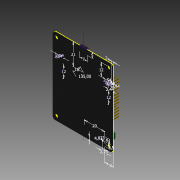
# Autodesk Inventor part: VeyronServoDriver
Saved by Autodesk Inventor 2015 (Build 190159000, 159)
## iProperties
Created: 2015-10-10
Part Number: VeyronServoDriver
Material: Generic
Document SubType Name: Modeling
Designer: styku
Density: 1 g/cm^3
Appearance: Default
Mass: 6.61804 g
Surface Area: 124.511 cm^2
Volume: 6.61804 cm^3
Author: styku
Autodesk Inventor part; units mm, degrees
ref_plane "YZ Plane" through (0, 0, 0) normal (1, 0, 0) x (0, 1, 0)
ref_plane "XZ Plane" through (0, 0, 0) normal (0, 1, 0) x (-1, 0, 0)
ref_plane "XY Plane" through (0, 0, 0) normal (0, 0, 1) x (1, 0, 0)
sketch "Sketch1" plane through (0, 0, 0) normal (0, 1, 0) x (-1, 0, 0)
  line L0 (22, 0) -> (-23, 0) construction
  line L1 (26.5, -36.5) -> (-26.5, -36.5)
  line L2 (-26.5, 36.5) -> (26.5, 36.5)
  line L3 (28.5, 34.5) -> (28.5, -34.5)
  line L4 (-28.5, -34.5) -> (-28.5, 34.5)
  line L5 (0, 32.6896) -> (0, -29) construction
  circle A0 centre (25, 32.5) radius 1.5
  circle A1 centre (-25, 32.5) radius 1.5
  circle A2 centre (25, -32.5) radius 1.5
  circle A3 centre (-25, -32.5) radius 1.5
  arc A4 (28.5, 34.5) -> (26.5, 36.5) centre (26.5, 34.5) ccw
  arc A5 (-26.5, 36.5) -> (-28.5, 34.5) centre (-26.5, 34.5) ccw
  arc A6 (-28.5, -34.5) -> (-26.5, -36.5) centre (-26.5, -34.5) ccw
  arc A7 (26.5, -36.5) -> (28.5, -34.5) centre (26.5, -34.5) ccw
  point P0 (0, 0)
  dimension "d1" = 73
  dimension "d2" = 57
  dimension "d3" = 3
  dimension "d4" = 32.5
  dimension "d5" = 25
  dimension "d6" = 2
  dimension "d7" = 2
  constraints: 12 end point, 8 centre point, 8 point on circle, 8 tangent, 3 symmetric about line, 2 equal radius, 2 horizontal, 2 vertical, 1 parallel, 5 other
  measures "d1" distance between parallel lines of L2 L1
  measures "d2" distance between parallel lines of L4 L3
  measures "d3" diameter of A0
  measures "d4" distance from line of L0 A0.centre
  measures "d5" distance from line of L5 A0.centre
  measures "d6" radius of A4
  measures "d7" radius of A5
extrude "Extrusion1" add sketch "Sketch1" along normal blind 1
sketch "Sketch2" plane through (0, 1, 0) normal (0, 1, 0) x (1, 0, 0)
  circle A0 centre (25, 32.5) radius 1.5 projected
  circle A1 centre (-25, 32.5) radius 1.5 projected
  circle A2 centre (25, -32.5) radius 1.5 projected
  circle A3 centre (-25, -32.5) radius 1.5 projected
  line L0 (-28.5, 34.5) -> (-28.5, -34.5) projected
  arc A4 (-28.5, -34.5) -> (-26.5, -36.5) centre (-26.5, -34.5) ccw projected
  line L1 (-26.5, -36.5) -> (26.5, -36.5) projected
  arc A5 (26.5, -36.5) -> (28.5, -34.5) centre (26.5, -34.5) ccw projected
  line L2 (28.5, -34.5) -> (28.5, 34.5) projected
  arc A6 (28.5, 34.5) -> (26.5, 36.5) centre (26.5, 34.5) ccw projected
  line L3 (26.5, 36.5) -> (-26.5, 36.5) projected
  arc A7 (-26.5, 36.5) -> (-28.5, 34.5) centre (-26.5, 34.5) ccw projected
  circle A8 centre (25, 32.5) radius 1.5 construction
  line L4 (24.06, -20.5) -> (26.5, -20.5)
  line L5 (26.5, -20.5) -> (26.5, -18.06)
  line L6 (26.5, -18.06) -> (24.06, -18.06)
  line L7 (24.06, -18.06) -> (24.06, -20.5)
  line L8 (22.2977, -19.28) -> (27.9142, -19.28) construction
  line L9 (25.28, -22.2473) -> (25.28, -16.4928) construction
  line L10 (24.96, -19.6) -> (25.6, -19.6)
  line L11 (25.6, -19.6) -> (25.6, -18.96)
  line L12 (25.6, -18.96) -> (24.96, -18.96)
  line L13 (24.96, -18.96) -> (24.96, -19.6)
  line L14 (24.06, -17.96) -> (26.5, -17.96)
  line L15 (26.5, -17.96) -> (26.5, -15.52)
  line L16 (26.5, -15.52) -> (24.06, -15.52)
  line L17 (24.06, -15.52) -> (24.06, -17.96)
  line L18 (24.96, -17.06) -> (25.6, -17.06)
  line L19 (25.6, -17.06) -> (25.6, -16.42)
  line L20 (25.6, -16.42) -> (24.96, -16.42)
  line L21 (24.96, -16.42) -> (24.96, -17.06)
  line L22 (24.06, -15.42) -> (26.5, -15.42)
  line L23 (26.5, -15.42) -> (26.5, -12.98)
  line L24 (26.5, -12.98) -> (24.06, -12.98)
  line L25 (24.06, -12.98) -> (24.06, -15.42)
  line L26 (24.96, -14.52) -> (25.6, -14.52)
  line L27 (25.6, -14.52) -> (25.6, -13.88)
  line L28 (25.6, -13.88) -> (24.96, -13.88)
  line L29 (24.96, -13.88) -> (24.96, -14.52)
  line L30 (24.06, -12.88) -> (26.5, -12.88)
  line L31 (26.5, -12.88) -> (26.5, -10.44)
  line L32 (26.5, -10.44) -> (24.06, -10.44)
  line L33 (24.06, -10.44) -> (24.06, -12.88)
  line L34 (24.96, -11.98) -> (25.6, -11.98)
  line L35 (25.6, -11.98) -> (25.6, -11.34)
  line L36 (25.6, -11.34) -> (24.96, -11.34)
  line L37 (24.96, -11.34) -> (24.96, -11.98)
  line L38 (21.52, -20.5) -> (23.96, -20.5)
  line L39 (23.96, -20.5) -> (23.96, -18.06)
  line L40 (23.96, -18.06) -> (21.52, -18.06)
  line L41 (21.52, -18.06) -> (21.52, -20.5)
  line L42 (22.42, -19.6) -> (23.06, -19.6)
  line L43 (23.06, -19.6) -> (23.06, -18.96)
  line L44 (23.06, -18.96) -> (22.42, -18.96)
  line L45 (22.42, -18.96) -> (22.42, -19.6)
  line L46 (21.52, -17.96) -> (23.96, -17.96)
  line L47 (23.96, -17.96) -> (23.96, -15.52)
  line L48 (23.96, -15.52) -> (21.52, -15.52)
  line L49 (21.52, -15.52) -> (21.52, -17.96)
  line L50 (22.42, -17.06) -> (23.06, -17.06)
  line L51 (23.06, -17.06) -> (23.06, -16.42)
  line L52 (23.06, -16.42) -> (22.42, -16.42)
  line L53 (22.42, -16.42) -> (22.42, -17.06)
  line L54 (21.52, -15.42) -> (23.96, -15.42)
  line L55 (23.96, -15.42) -> (23.96, -12.98)
  line L56 (23.96, -12.98) -> (21.52, -12.98)
  line L57 (21.52, -12.98) -> (21.52, -15.42)
  line L58 (22.42, -14.52) -> (23.06, -14.52)
  line L59 (23.06, -14.52) -> (23.06, -13.88)
  line L60 (23.06, -13.88) -> (22.42, -13.88)
  line L61 (22.42, -13.88) -> (22.42, -14.52)
  line L62 (21.52, -12.88) -> (23.96, -12.88)
  line L63 (23.96, -12.88) -> (23.96, -10.44)
  line L64 (23.96, -10.44) -> (21.52, -10.44)
  line L65 (21.52, -10.44) -> (21.52, -12.88)
  line L66 (22.42, -11.98) -> (23.06, -11.98)
  line L67 (23.06, -11.98) -> (23.06, -11.34)
  line L68 (23.06, -11.34) -> (22.42, -11.34)
  line L69 (22.42, -11.34) -> (22.42, -11.98)
  line L70 (18.98, -20.5) -> (21.42, -20.5)
  line L71 (21.42, -20.5) -> (21.42, -18.06)
  line L72 (21.42, -18.06) -> (18.98, -18.06)
  line L73 (18.98, -18.06) -> (18.98, -20.5)
  line L74 (19.88, -19.6) -> (20.52, -19.6)
  line L75 (20.52, -19.6) -> (20.52, -18.96)
  line L76 (20.52, -18.96) -> (19.88, -18.96)
  line L77 (19.88, -18.96) -> (19.88, -19.6)
  line L78 (18.98, -17.96) -> (21.42, -17.96)
  line L79 (21.42, -17.96) -> (21.42, -15.52)
  line L80 (21.42, -15.52) -> (18.98, -15.52)
  line L81 (18.98, -15.52) -> (18.98, -17.96)
  line L82 (19.88, -17.06) -> (20.52, -17.06)
  line L83 (20.52, -17.06) -> (20.52, -16.42)
  line L84 (20.52, -16.42) -> (19.88, -16.42)
  line L85 (19.88, -16.42) -> (19.88, -17.06)
  line L86 (18.98, -15.42) -> (21.42, -15.42)
  line L87 (21.42, -15.42) -> (21.42, -12.98)
  line L88 (21.42, -12.98) -> (18.98, -12.98)
  line L89 (18.98, -12.98) -> (18.98, -15.42)
  line L90 (19.88, -14.52) -> (20.52, -14.52)
  line L91 (20.52, -14.52) -> (20.52, -13.88)
  line L92 (20.52, -13.88) -> (19.88, -13.88)
  line L93 (19.88, -13.88) -> (19.88, -14.52)
  line L94 (18.98, -12.88) -> (21.42, -12.88)
  line L95 (21.42, -12.88) -> (21.42, -10.44)
  line L96 (21.42, -10.44) -> (18.98, -10.44)
  line L97 (18.98, -10.44) -> (18.98, -12.88)
  line L98 (19.88, -11.98) -> (20.52, -11.98)
  line L99 (20.52, -11.98) -> (20.52, -11.34)
  line L100 (20.52, -11.34) -> (19.88, -11.34)
  line L101 (19.88, -11.34) -> (19.88, -11.98)
  line L102 (24.06, -8.5) -> (26.5, -8.5)
  line L103 (26.5, -8.5) -> (26.5, -6.06)
  line L104 (26.5, -6.06) -> (24.06, -6.06)
  line L105 (24.06, -6.06) -> (24.06, -8.5)
  line L106 (22.2977, -7.28) -> (27.9142, -7.28) construction
  line L107 (25.28, -10.2473) -> (25.28, -4.4928) construction
  line L108 (24.96, -7.6) -> (25.6, -7.6)
  line L109 (25.6, -7.6) -> (25.6, -6.96)
  line L110 (25.6, -6.96) -> (24.96, -6.96)
  line L111 (24.96, -6.96) -> (24.96, -7.6)
  line L112 (24.06, -5.96) -> (26.5, -5.96)
  line L113 (26.5, -5.96) -> (26.5, -3.52)
  line L114 (24.06, -3.52) -> (24.06, -5.96)
  line L115 (26.5, -3.52) -> (24.06, -3.52)
  line L116 (25.6, -4.42) -> (24.96, -4.42)
  line L117 (24.96, -4.42) -> (24.96, -5.06)
  line L118 (24.96, -5.06) -> (25.6, -5.06)
  line L119 (25.6, -5.06) -> (25.6, -4.42)
  line L120 (24.06, -3.42) -> (26.5, -3.42)
  line L121 (26.5, -3.42) -> (26.5, -0.98)
  line L122 (24.06, -0.98) -> (24.06, -3.42)
  line L123 (26.5, -0.98) -> (24.06, -0.98)
  line L124 (25.6, -1.88) -> (24.96, -1.88)
  line L125 (24.96, -1.88) -> (24.96, -2.52)
  line L126 (24.96, -2.52) -> (25.6, -2.52)
  line L127 (25.6, -2.52) -> (25.6, -1.88)
  line L128 (24.06, -0.88) -> (26.5, -0.88)
  line L129 (26.5, -0.88) -> (26.5, 1.56)
  line L130 (24.06, 1.56) -> (24.06, -0.88)
  line L131 (26.5, 1.56) -> (24.06, 1.56)
  line L132 (25.6, 0.66) -> (24.96, 0.66)
  line L133 (24.96, 0.66) -> (24.96, 0.02)
  line L134 (24.96, 0.02) -> (25.6, 0.02)
  line L135 (25.6, 0.02) -> (25.6, 0.66)
  line L136 (21.52, -8.5) -> (23.96, -8.5)
  line L137 (23.96, -8.5) -> (23.96, -6.06)
  line L138 (21.52, -6.06) -> (21.52, -8.5)
  line L139 (23.96, -6.06) -> (21.52, -6.06)
  line L140 (23.06, -6.96) -> (22.42, -6.96)
  line L141 (22.42, -6.96) -> (22.42, -7.6)
  line L142 (22.42, -7.6) -> (23.06, -7.6)
  line L143 (23.06, -7.6) -> (23.06, -6.96)
  line L144 (21.52, -5.96) -> (23.96, -5.96)
  line L145 (23.96, -5.96) -> (23.96, -3.52)
  line L146 (21.52, -3.52) -> (21.52, -5.96)
  line L147 (23.96, -3.52) -> (21.52, -3.52)
  line L148 (23.06, -4.42) -> (22.42, -4.42)
  line L149 (22.42, -4.42) -> (22.42, -5.06)
  line L150 (22.42, -5.06) -> (23.06, -5.06)
  line L151 (23.06, -5.06) -> (23.06, -4.42)
  line L152 (21.52, -3.42) -> (23.96, -3.42)
  line L153 (23.96, -3.42) -> (23.96, -0.98)
  line L154 (21.52, -0.98) -> (21.52, -3.42)
  line L155 (23.96, -0.98) -> (21.52, -0.98)
  line L156 (23.06, -1.88) -> (22.42, -1.88)
  line L157 (22.42, -1.88) -> (22.42, -2.52)
  line L158 (22.42, -2.52) -> (23.06, -2.52)
  line L159 (23.06, -2.52) -> (23.06, -1.88)
  line L160 (21.52, -0.88) -> (23.96, -0.88)
  line L161 (23.96, -0.88) -> (23.96, 1.56)
  line L162 (21.52, 1.56) -> (21.52, -0.88)
  line L163 (23.96, 1.56) -> (21.52, 1.56)
  line L164 (23.06, 0.66) -> (22.42, 0.66)
  line L165 (22.42, 0.66) -> (22.42, 0.02)
  line L166 (22.42, 0.02) -> (23.06, 0.02)
  line L167 (23.06, 0.02) -> (23.06, 0.66)
  line L168 (18.98, -8.5) -> (21.42, -8.5)
  line L169 (21.42, -8.5) -> (21.42, -6.06)
  line L170 (18.98, -6.06) -> (18.98, -8.5)
  line L171 (21.42, -6.06) -> (18.98, -6.06)
  line L172 (20.52, -6.96) -> (19.88, -6.96)
  line L173 (19.88, -6.96) -> (19.88, -7.6)
  line L174 (19.88, -7.6) -> (20.52, -7.6)
  line L175 (20.52, -7.6) -> (20.52, -6.96)
  line L176 (18.98, -5.96) -> (21.42, -5.96)
  line L177 (21.42, -5.96) -> (21.42, -3.52)
  line L178 (18.98, -3.52) -> (18.98, -5.96)
  line L179 (21.42, -3.52) -> (18.98, -3.52)
  line L180 (20.52, -4.42) -> (19.88, -4.42)
  line L181 (19.88, -4.42) -> (19.88, -5.06)
  line L182 (19.88, -5.06) -> (20.52, -5.06)
  line L183 (20.52, -5.06) -> (20.52, -4.42)
  line L184 (18.98, -3.42) -> (21.42, -3.42)
  line L185 (21.42, -3.42) -> (21.42, -0.98)
  line L186 (18.98, -0.98) -> (18.98, -3.42)
  line L187 (21.42, -0.98) -> (18.98, -0.98)
  line L188 (20.52, -1.88) -> (19.88, -1.88)
  line L189 (19.88, -1.88) -> (19.88, -2.52)
  line L190 (19.88, -2.52) -> (20.52, -2.52)
  line L191 (20.52, -2.52) -> (20.52, -1.88)
  line L192 (18.98, -0.88) -> (21.42, -0.88)
  line L193 (21.42, -0.88) -> (21.42, 1.56)
  line L194 (18.98, 1.56) -> (18.98, -0.88)
  line L195 (21.42, 1.56) -> (18.98, 1.56)
  line L196 (20.52, 0.66) -> (19.88, 0.66)
  line L197 (19.88, 0.66) -> (19.88, 0.02)
  line L198 (19.88, 0.02) -> (20.52, 0.02)
  line L199 (20.52, 0.02) -> (20.52, 0.66)
  line L200 (24.06, 3.5) -> (26.5, 3.5)
  line L201 (26.5, 3.5) -> (26.5, 5.94)
  line L202 (26.5, 5.94) -> (24.06, 5.94)
  line L203 (24.06, 5.94) -> (24.06, 3.5)
  line L204 (22.2977, 4.72) -> (27.9142, 4.72) construction
  line L205 (25.28, 1.7527) -> (25.28, 7.5072) construction
  line L206 (24.96, 4.4) -> (25.6, 4.4)
  line L207 (25.6, 4.4) -> (25.6, 5.04)
  line L208 (25.6, 5.04) -> (24.96, 5.04)
  line L209 (24.96, 5.04) -> (24.96, 4.4)
  line L210 (24.06, 6.04) -> (26.5, 6.04)
  line L211 (26.5, 6.04) -> (26.5, 8.48)
  line L212 (24.06, 8.48) -> (24.06, 6.04)
  line L213 (26.5, 8.48) -> (24.06, 8.48)
  line L214 (25.6, 7.58) -> (24.96, 7.58)
  line L215 (24.96, 7.58) -> (24.96, 6.94)
  line L216 (24.96, 6.94) -> (25.6, 6.94)
  line L217 (25.6, 6.94) -> (25.6, 7.58)
  line L218 (24.06, 8.58) -> (26.5, 8.58)
  line L219 (26.5, 8.58) -> (26.5, 11.02)
  line L220 (24.06, 11.02) -> (24.06, 8.58)
  line L221 (26.5, 11.02) -> (24.06, 11.02)
  line L222 (25.6, 10.12) -> (24.96, 10.12)
  line L223 (24.96, 10.12) -> (24.96, 9.48)
  line L224 (24.96, 9.48) -> (25.6, 9.48)
  line L225 (25.6, 9.48) -> (25.6, 10.12)
  line L226 (24.06, 11.12) -> (26.5, 11.12)
  line L227 (26.5, 11.12) -> (26.5, 13.56)
  line L228 (24.06, 13.56) -> (24.06, 11.12)
  line L229 (26.5, 13.56) -> (24.06, 13.56)
  line L230 (25.6, 12.66) -> (24.96, 12.66)
  line L231 (24.96, 12.66) -> (24.96, 12.02)
  line L232 (24.96, 12.02) -> (25.6, 12.02)
  line L233 (25.6, 12.02) -> (25.6, 12.66)
  line L234 (21.52, 3.5) -> (23.96, 3.5)
  line L235 (23.96, 3.5) -> (23.96, 5.94)
  line L236 (21.52, 5.94) -> (21.52, 3.5)
  line L237 (23.96, 5.94) -> (21.52, 5.94)
  line L238 (23.06, 5.04) -> (22.42, 5.04)
  line L239 (22.42, 5.04) -> (22.42, 4.4)
  line L240 (22.42, 4.4) -> (23.06, 4.4)
  line L241 (23.06, 4.4) -> (23.06, 5.04)
  line L242 (21.52, 6.04) -> (23.96, 6.04)
  line L243 (23.96, 6.04) -> (23.96, 8.48)
  line L244 (21.52, 8.48) -> (21.52, 6.04)
  line L245 (23.96, 8.48) -> (21.52, 8.48)
  line L246 (23.06, 7.58) -> (22.42, 7.58)
  line L247 (22.42, 7.58) -> (22.42, 6.94)
  line L248 (22.42, 6.94) -> (23.06, 6.94)
  line L249 (23.06, 6.94) -> (23.06, 7.58)
  line L250 (21.52, 8.58) -> (23.96, 8.58)
  line L251 (23.96, 8.58) -> (23.96, 11.02)
  line L252 (21.52, 11.02) -> (21.52, 8.58)
  line L253 (23.96, 11.02) -> (21.52, 11.02)
  line L254 (23.06, 10.12) -> (22.42, 10.12)
  line L255 (22.42, 10.12) -> (22.42, 9.48)
  line L256 (22.42, 9.48) -> (23.06, 9.48)
  line L257 (23.06, 9.48) -> (23.06, 10.12)
  line L258 (21.52, 11.12) -> (23.96, 11.12)
  line L259 (23.96, 11.12) -> (23.96, 13.56)
  line L260 (21.52, 13.56) -> (21.52, 11.12)
  line L261 (23.96, 13.56) -> (21.52, 13.56)
  line L262 (23.06, 12.66) -> (22.42, 12.66)
  line L263 (22.42, 12.66) -> (22.42, 12.02)
  line L264 (22.42, 12.02) -> (23.06, 12.02)
  line L265 (23.06, 12.02) -> (23.06, 12.66)
  line L266 (18.98, 3.5) -> (21.42, 3.5)
  line L267 (21.42, 3.5) -> (21.42, 5.94)
  line L268 (18.98, 5.94) -> (18.98, 3.5)
  line L269 (21.42, 5.94) -> (18.98, 5.94)
  line L270 (20.52, 5.04) -> (19.88, 5.04)
  line L271 (19.88, 5.04) -> (19.88, 4.4)
  line L272 (19.88, 4.4) -> (20.52, 4.4)
  line L273 (20.52, 4.4) -> (20.52, 5.04)
  line L274 (18.98, 6.04) -> (21.42, 6.04)
  line L275 (21.42, 6.04) -> (21.42, 8.48)
  line L276 (18.98, 8.48) -> (18.98, 6.04)
  line L277 (21.42, 8.48) -> (18.98, 8.48)
  line L278 (20.52, 7.58) -> (19.88, 7.58)
  line L279 (19.88, 7.58) -> (19.88, 6.94)
  line L280 (19.88, 6.94) -> (20.52, 6.94)
  line L281 (20.52, 6.94) -> (20.52, 7.58)
  line L282 (18.98, 8.58) -> (21.42, 8.58)
  line L283 (21.42, 8.58) -> (21.42, 11.02)
  line L284 (18.98, 11.02) -> (18.98, 8.58)
  line L285 (21.42, 11.02) -> (18.98, 11.02)
  line L286 (20.52, 10.12) -> (19.88, 10.12)
  line L287 (19.88, 10.12) -> (19.88, 9.48)
  line L288 (19.88, 9.48) -> (20.52, 9.48)
  line L289 (20.52, 9.48) -> (20.52, 10.12)
  line L290 (18.98, 11.12) -> (21.42, 11.12)
  line L291 (21.42, 11.12) -> (21.42, 13.56)
  line L292 (18.98, 13.56) -> (18.98, 11.12)
  line L293 (21.42, 13.56) -> (18.98, 13.56)
  line L294 (20.52, 12.66) -> (19.88, 12.66)
  line L295 (19.88, 12.66) -> (19.88, 12.02)
  line L296 (19.88, 12.02) -> (20.52, 12.02)
  line L297 (20.52, 12.02) -> (20.52, 12.66)
  line L298 (0, 41) -> (0, -49) construction
  line L299 (-24.06, -20.5) -> (-26.5, -20.5)
  line L300 (-26.5, -20.5) -> (-26.5, -18.06)
  line L301 (-26.5, -18.06) -> (-24.06, -18.06)
  line L302 (-24.06, -18.06) -> (-24.06, -20.5)
  line L303 (-24.96, -19.6) -> (-25.6, -19.6)
  line L304 (-25.6, -19.6) -> (-25.6, -18.96)
  line L305 (-25.6, -18.96) -> (-24.96, -18.96)
  line L306 (-24.96, -18.96) -> (-24.96, -19.6)
  line L307 (-24.06, -17.96) -> (-26.5, -17.96)
  line L308 (-26.5, -17.96) -> (-26.5, -15.52)
  line L309 (-26.5, -15.52) -> (-24.06, -15.52)
  line L310 (-24.06, -15.52) -> (-24.06, -17.96)
  line L311 (-24.96, -17.06) -> (-25.6, -17.06)
  line L312 (-25.6, -17.06) -> (-25.6, -16.42)
  line L313 (-25.6, -16.42) -> (-24.96, -16.42)
  line L314 (-24.96, -16.42) -> (-24.96, -17.06)
  line L315 (-24.06, -15.42) -> (-26.5, -15.42)
  line L316 (-26.5, -15.42) -> (-26.5, -12.98)
  line L317 (-26.5, -12.98) -> (-24.06, -12.98)
  line L318 (-24.06, -12.98) -> (-24.06, -15.42)
  line L319 (-24.96, -14.52) -> (-25.6, -14.52)
  line L320 (-25.6, -14.52) -> (-25.6, -13.88)
  line L321 (-25.6, -13.88) -> (-24.96, -13.88)
  line L322 (-24.96, -13.88) -> (-24.96, -14.52)
  line L323 (-24.06, -12.88) -> (-26.5, -12.88)
  line L324 (-26.5, -12.88) -> (-26.5, -10.44)
  line L325 (-26.5, -10.44) -> (-24.06, -10.44)
  line L326 (-24.06, -10.44) -> (-24.06, -12.88)
  line L327 (-24.96, -11.98) -> (-25.6, -11.98)
  line L328 (-25.6, -11.98) -> (-25.6, -11.34)
  line L329 (-25.6, -11.34) -> (-24.96, -11.34)
  line L330 (-24.96, -11.34) -> (-24.96, -11.98)
  line L331 (-21.52, -20.5) -> (-23.96, -20.5)
  line L332 (-23.96, -20.5) -> (-23.96, -18.06)
  line L333 (-23.96, -18.06) -> (-21.52, -18.06)
  line L334 (-21.52, -18.06) -> (-21.52, -20.5)
  line L335 (-22.42, -19.6) -> (-23.06, -19.6)
  line L336 (-23.06, -19.6) -> (-23.06, -18.96)
  line L337 (-23.06, -18.96) -> (-22.42, -18.96)
  line L338 (-22.42, -18.96) -> (-22.42, -19.6)
  line L339 (-21.52, -17.96) -> (-23.96, -17.96)
  line L340 (-23.96, -17.96) -> (-23.96, -15.52)
  line L341 (-23.96, -15.52) -> (-21.52, -15.52)
  line L342 (-21.52, -15.52) -> (-21.52, -17.96)
  line L343 (-22.42, -17.06) -> (-23.06, -17.06)
  line L344 (-23.06, -17.06) -> (-23.06, -16.42)
  line L345 (-23.06, -16.42) -> (-22.42, -16.42)
  line L346 (-22.42, -16.42) -> (-22.42, -17.06)
  line L347 (-21.52, -15.42) -> (-23.96, -15.42)
  line L348 (-23.96, -15.42) -> (-23.96, -12.98)
  line L349 (-23.96, -12.98) -> (-21.52, -12.98)
  line L350 (-21.52, -12.98) -> (-21.52, -15.42)
  line L351 (-22.42, -14.52) -> (-23.06, -14.52)
  line L352 (-23.06, -14.52) -> (-23.06, -13.88)
  line L353 (-23.06, -13.88) -> (-22.42, -13.88)
  line L354 (-22.42, -13.88) -> (-22.42, -14.52)
  line L355 (-21.52, -12.88) -> (-23.96, -12.88)
  line L356 (-23.96, -12.88) -> (-23.96, -10.44)
  line L357 (-23.96, -10.44) -> (-21.52, -10.44)
  line L358 (-21.52, -10.44) -> (-21.52, -12.88)
  line L359 (-22.42, -11.98) -> (-23.06, -11.98)
  line L360 (-23.06, -11.98) -> (-23.06, -11.34)
  line L361 (-23.06, -11.34) -> (-22.42, -11.34)
  line L362 (-22.42, -11.34) -> (-22.42, -11.98)
  line L363 (-18.98, -20.5) -> (-21.42, -20.5)
  line L364 (-21.42, -20.5) -> (-21.42, -18.06)
  line L365 (-21.42, -18.06) -> (-18.98, -18.06)
  line L366 (-18.98, -18.06) -> (-18.98, -20.5)
  line L367 (-19.88, -19.6) -> (-20.52, -19.6)
  line L368 (-20.52, -19.6) -> (-20.52, -18.96)
  line L369 (-20.52, -18.96) -> (-19.88, -18.96)
  line L370 (-19.88, -18.96) -> (-19.88, -19.6)
  line L371 (-18.98, -17.96) -> (-21.42, -17.96)
  line L372 (-21.42, -17.96) -> (-21.42, -15.52)
  line L373 (-21.42, -15.52) -> (-18.98, -15.52)
  line L374 (-18.98, -15.52) -> (-18.98, -17.96)
  line L375 (-19.88, -17.06) -> (-20.52, -17.06)
  line L376 (-20.52, -17.06) -> (-20.52, -16.42)
  line L377 (-20.52, -16.42) -> (-19.88, -16.42)
  line L378 (-19.88, -16.42) -> (-19.88, -17.06)
  line L379 (-18.98, -15.42) -> (-21.42, -15.42)
  line L380 (-21.42, -15.42) -> (-21.42, -12.98)
  line L381 (-21.42, -12.98) -> (-18.98, -12.98)
  line L382 (-18.98, -12.98) -> (-18.98, -15.42)
  line L383 (-19.88, -14.52) -> (-20.52, -14.52)
  line L384 (-20.52, -14.52) -> (-20.52, -13.88)
  line L385 (-20.52, -13.88) -> (-19.88, -13.88)
  line L386 (-19.88, -13.88) -> (-19.88, -14.52)
  line L387 (-18.98, -12.88) -> (-21.42, -12.88)
  line L388 (-21.42, -12.88) -> (-21.42, -10.44)
  line L389 (-21.42, -10.44) -> (-18.98, -10.44)
  line L390 (-18.98, -10.44) -> (-18.98, -12.88)
  line L391 (-19.88, -11.98) -> (-20.52, -11.98)
  line L392 (-20.52, -11.98) -> (-20.52, -11.34)
  line L393 (-20.52, -11.34) -> (-19.88, -11.34)
  line L394 (-19.88, -11.34) -> (-19.88, -11.98)
  line L395 (-24.06, -8.5) -> (-26.5, -8.5)
  line L396 (-26.5, -8.5) -> (-26.5, -6.06)
  line L397 (-26.5, -6.06) -> (-24.06, -6.06)
  line L398 (-24.06, -6.06) -> (-24.06, -8.5)
  line L399 (-24.96, -7.6) -> (-25.6, -7.6)
  line L400 (-25.6, -7.6) -> (-25.6, -6.96)
  line L401 (-25.6, -6.96) -> (-24.96, -6.96)
  line L402 (-24.96, -6.96) -> (-24.96, -7.6)
  line L403 (-26.5, -3.52) -> (-24.06, -3.52)
  line L404 (-24.96, -4.42) -> (-24.96, -5.06)
  line L405 (-24.96, -5.06) -> (-25.6, -5.06)
  line L406 (-25.6, -5.06) -> (-25.6, -4.42)
  line L407 (-24.06, -5.96) -> (-26.5, -5.96)
  line L408 (-26.5, -5.96) -> (-26.5, -3.52)
  line L409 (-24.06, -3.52) -> (-24.06, -5.96)
  line L410 (-25.6, -4.42) -> (-24.96, -4.42)
  line L411 (-26.5, -0.98) -> (-24.06, -0.98)
  line L412 (-24.96, -1.88) -> (-24.96, -2.52)
  line L413 (-24.96, -2.52) -> (-25.6, -2.52)
  line L414 (-25.6, -2.52) -> (-25.6, -1.88)
  line L415 (-24.06, -3.42) -> (-26.5, -3.42)
  line L416 (-26.5, -3.42) -> (-26.5, -0.98)
  line L417 (-24.06, -0.98) -> (-24.06, -3.42)
  line L418 (-25.6, -1.88) -> (-24.96, -1.88)
  line L419 (-26.5, 1.56) -> (-24.06, 1.56)
  line L420 (-24.96, 0.66) -> (-24.96, 0.02)
  line L421 (-24.96, 0.02) -> (-25.6, 0.02)
  line L422 (-25.6, 0.02) -> (-25.6, 0.66)
  line L423 (-24.06, -0.88) -> (-26.5, -0.88)
  line L424 (-26.5, -0.88) -> (-26.5, 1.56)
  line L425 (-24.06, 1.56) -> (-24.06, -0.88)
  line L426 (-25.6, 0.66) -> (-24.96, 0.66)
  line L427 (-23.96, -6.06) -> (-21.52, -6.06)
  line L428 (-22.42, -6.96) -> (-22.42, -7.6)
  line L429 (-22.42, -7.6) -> (-23.06, -7.6)
  line L430 (-23.06, -7.6) -> (-23.06, -6.96)
  line L431 (-21.52, -8.5) -> (-23.96, -8.5)
  line L432 (-23.96, -8.5) -> (-23.96, -6.06)
  line L433 (-21.52, -6.06) -> (-21.52, -8.5)
  line L434 (-23.06, -6.96) -> (-22.42, -6.96)
  line L435 (-23.96, -3.52) -> (-21.52, -3.52)
  line L436 (-22.42, -4.42) -> (-22.42, -5.06)
  line L437 (-22.42, -5.06) -> (-23.06, -5.06)
  line L438 (-23.06, -5.06) -> (-23.06, -4.42)
  line L439 (-21.52, -5.96) -> (-23.96, -5.96)
  line L440 (-23.96, -5.96) -> (-23.96, -3.52)
  line L441 (-21.52, -3.52) -> (-21.52, -5.96)
  line L442 (-23.06, -4.42) -> (-22.42, -4.42)
  line L443 (-23.96, -0.98) -> (-21.52, -0.98)
  line L444 (-22.42, -1.88) -> (-22.42, -2.52)
  line L445 (-22.42, -2.52) -> (-23.06, -2.52)
  line L446 (-23.06, -2.52) -> (-23.06, -1.88)
  line L447 (-21.52, -3.42) -> (-23.96, -3.42)
  line L448 (-23.96, -3.42) -> (-23.96, -0.98)
  line L449 (-21.52, -0.98) -> (-21.52, -3.42)
  line L450 (-23.06, -1.88) -> (-22.42, -1.88)
  line L451 (-23.96, 1.56) -> (-21.52, 1.56)
  line L452 (-22.42, 0.66) -> (-22.42, 0.02)
  line L453 (-22.42, 0.02) -> (-23.06, 0.02)
  line L454 (-23.06, 0.02) -> (-23.06, 0.66)
  line L455 (-21.52, -0.88) -> (-23.96, -0.88)
  line L456 (-23.96, -0.88) -> (-23.96, 1.56)
  line L457 (-21.52, 1.56) -> (-21.52, -0.88)
  line L458 (-23.06, 0.66) -> (-22.42, 0.66)
  line L459 (-21.42, -6.06) -> (-18.98, -6.06)
  line L460 (-19.88, -6.96) -> (-19.88, -7.6)
  line L461 (-19.88, -7.6) -> (-20.52, -7.6)
  line L462 (-20.52, -7.6) -> (-20.52, -6.96)
  line L463 (-18.98, -8.5) -> (-21.42, -8.5)
  line L464 (-21.42, -8.5) -> (-21.42, -6.06)
  line L465 (-18.98, -6.06) -> (-18.98, -8.5)
  line L466 (-20.52, -6.96) -> (-19.88, -6.96)
  line L467 (-21.42, -3.52) -> (-18.98, -3.52)
  line L468 (-19.88, -4.42) -> (-19.88, -5.06)
  line L469 (-19.88, -5.06) -> (-20.52, -5.06)
  line L470 (-20.52, -5.06) -> (-20.52, -4.42)
  line L471 (-18.98, -5.96) -> (-21.42, -5.96)
  line L472 (-21.42, -5.96) -> (-21.42, -3.52)
  line L473 (-18.98, -3.52) -> (-18.98, -5.96)
  line L474 (-20.52, -4.42) -> (-19.88, -4.42)
  line L475 (-21.42, -0.98) -> (-18.98, -0.98)
  line L476 (-19.88, -1.88) -> (-19.88, -2.52)
  line L477 (-19.88, -2.52) -> (-20.52, -2.52)
  line L478 (-20.52, -2.52) -> (-20.52, -1.88)
  line L479 (-18.98, -3.42) -> (-21.42, -3.42)
  line L480 (-21.42, -3.42) -> (-21.42, -0.98)
  line L481 (-18.98, -0.98) -> (-18.98, -3.42)
  line L482 (-20.52, -1.88) -> (-19.88, -1.88)
  line L483 (-21.42, 1.56) -> (-18.98, 1.56)
  line L484 (-19.88, 0.66) -> (-19.88, 0.02)
  line L485 (-19.88, 0.02) -> (-20.52, 0.02)
  line L486 (-20.52, 0.02) -> (-20.52, 0.66)
  line L487 (-18.98, -0.88) -> (-21.42, -0.88)
  line L488 (-21.42, -0.88) -> (-21.42, 1.56)
  line L489 (-18.98, 1.56) -> (-18.98, -0.88)
  line L490 (-20.52, 0.66) -> (-19.88, 0.66)
  line L491 (-24.06, 3.5) -> (-26.5, 3.5)
  line L492 (-26.5, 3.5) -> (-26.5, 5.94)
  line L493 (-26.5, 5.94) -> (-24.06, 5.94)
  line L494 (-24.06, 5.94) -> (-24.06, 3.5)
  line L495 (-24.96, 4.4) -> (-25.6, 4.4)
  line L496 (-25.6, 4.4) -> (-25.6, 5.04)
  line L497 (-25.6, 5.04) -> (-24.96, 5.04)
  line L498 (-24.96, 5.04) -> (-24.96, 4.4)
  line L499 (-26.5, 8.48) -> (-24.06, 8.48)
  line L500 (-24.96, 7.58) -> (-24.96, 6.94)
  line L501 (-24.96, 6.94) -> (-25.6, 6.94)
  line L502 (-25.6, 6.94) -> (-25.6, 7.58)
  line L503 (-24.06, 6.04) -> (-26.5, 6.04)
  line L504 (-26.5, 6.04) -> (-26.5, 8.48)
  line L505 (-24.06, 8.48) -> (-24.06, 6.04)
  line L506 (-25.6, 7.58) -> (-24.96, 7.58)
  line L507 (-26.5, 11.02) -> (-24.06, 11.02)
  line L508 (-24.96, 10.12) -> (-24.96, 9.48)
  line L509 (-24.96, 9.48) -> (-25.6, 9.48)
  line L510 (-25.6, 9.48) -> (-25.6, 10.12)
  line L511 (-24.06, 8.58) -> (-26.5, 8.58)
  line L512 (-26.5, 8.58) -> (-26.5, 11.02)
  line L513 (-24.06, 11.02) -> (-24.06, 8.58)
  line L514 (-25.6, 10.12) -> (-24.96, 10.12)
  line L515 (-26.5, 13.56) -> (-24.06, 13.56)
  line L516 (-24.96, 12.66) -> (-24.96, 12.02)
  line L517 (-24.96, 12.02) -> (-25.6, 12.02)
  line L518 (-25.6, 12.02) -> (-25.6, 12.66)
  line L519 (-24.06, 11.12) -> (-26.5, 11.12)
  line L520 (-26.5, 11.12) -> (-26.5, 13.56)
  line L521 (-24.06, 13.56) -> (-24.06, 11.12)
  line L522 (-25.6, 12.66) -> (-24.96, 12.66)
  line L523 (-23.96, 5.94) -> (-21.52, 5.94)
  line L524 (-22.42, 5.04) -> (-22.42, 4.4)
  line L525 (-22.42, 4.4) -> (-23.06, 4.4)
  line L526 (-23.06, 4.4) -> (-23.06, 5.04)
  line L527 (-21.52, 3.5) -> (-23.96, 3.5)
  line L528 (-23.96, 3.5) -> (-23.96, 5.94)
  line L529 (-21.52, 5.94) -> (-21.52, 3.5)
  line L530 (-23.06, 5.04) -> (-22.42, 5.04)
  line L531 (-23.96, 8.48) -> (-21.52, 8.48)
  line L532 (-22.42, 7.58) -> (-22.42, 6.94)
  line L533 (-22.42, 6.94) -> (-23.06, 6.94)
  line L534 (-23.06, 6.94) -> (-23.06, 7.58)
  line L535 (-21.52, 6.04) -> (-23.96, 6.04)
  line L536 (-23.96, 6.04) -> (-23.96, 8.48)
  line L537 (-21.52, 8.48) -> (-21.52, 6.04)
  line L538 (-23.06, 7.58) -> (-22.42, 7.58)
  line L539 (-23.96, 11.02) -> (-21.52, 11.02)
  line L540 (-22.42, 10.12) -> (-22.42, 9.48)
  line L541 (-22.42, 9.48) -> (-23.06, 9.48)
  line L542 (-23.06, 9.48) -> (-23.06, 10.12)
  line L543 (-21.52, 8.58) -> (-23.96, 8.58)
  line L544 (-23.96, 8.58) -> (-23.96, 11.02)
  line L545 (-21.52, 11.02) -> (-21.52, 8.58)
  line L546 (-23.06, 10.12) -> (-22.42, 10.12)
  line L547 (-23.96, 13.56) -> (-21.52, 13.56)
  line L548 (-22.42, 12.66) -> (-22.42, 12.02)
  line L549 (-22.42, 12.02) -> (-23.06, 12.02)
  line L550 (-23.06, 12.02) -> (-23.06, 12.66)
  line L551 (-21.52, 11.12) -> (-23.96, 11.12)
  line L552 (-23.96, 11.12) -> (-23.96, 13.56)
  line L553 (-21.52, 13.56) -> (-21.52, 11.12)
  line L554 (-23.06, 12.66) -> (-22.42, 12.66)
  line L555 (-21.42, 5.94) -> (-18.98, 5.94)
  line L556 (-19.88, 5.04) -> (-19.88, 4.4)
  line L557 (-19.88, 4.4) -> (-20.52, 4.4)
  line L558 (-20.52, 4.4) -> (-20.52, 5.04)
  line L559 (-18.98, 3.5) -> (-21.42, 3.5)
  line L560 (-21.42, 3.5) -> (-21.42, 5.94)
  line L561 (-18.98, 5.94) -> (-18.98, 3.5)
  line L562 (-20.52, 5.04) -> (-19.88, 5.04)
  line L563 (-21.42, 8.48) -> (-18.98, 8.48)
  line L564 (-19.88, 7.58) -> (-19.88, 6.94)
  line L565 (-19.88, 6.94) -> (-20.52, 6.94)
  line L566 (-20.52, 6.94) -> (-20.52, 7.58)
  line L567 (-18.98, 6.04) -> (-21.42, 6.04)
  line L568 (-21.42, 6.04) -> (-21.42, 8.48)
  line L569 (-18.98, 8.48) -> (-18.98, 6.04)
  line L570 (-20.52, 7.58) -> (-19.88, 7.58)
  line L571 (-21.42, 11.02) -> (-18.98, 11.02)
  line L572 (-19.88, 10.12) -> (-19.88, 9.48)
  line L573 (-19.88, 9.48) -> (-20.52, 9.48)
  line L574 (-20.52, 9.48) -> (-20.52, 10.12)
  line L575 (-18.98, 8.58) -> (-21.42, 8.58)
  line L576 (-21.42, 8.58) -> (-21.42, 11.02)
  line L577 (-18.98, 11.02) -> (-18.98, 8.58)
  line L578 (-20.52, 10.12) -> (-19.88, 10.12)
  line L579 (-21.42, 13.56) -> (-18.98, 13.56)
  line L580 (-19.88, 12.66) -> (-19.88, 12.02)
  line L581 (-19.88, 12.02) -> (-20.52, 12.02)
  line L582 (-20.52, 12.02) -> (-20.52, 12.66)
  line L583 (-18.98, 11.12) -> (-21.42, 11.12)
  line L584 (-21.42, 11.12) -> (-21.42, 13.56)
  line L585 (-18.98, 13.56) -> (-18.98, 11.12)
  line L586 (-20.52, 12.66) -> (-19.88, 12.66)
  line L587 (0, -15.5) -> (-7.0711, -8.4289)
  line L588 (0, -15.5) -> (10, -15.5) construction
  line L589 (-7.0711, -8.4289) -> (0, -1.3579)
  line L590 (7.0711, -8.4289) -> (0, -15.5)
  line L591 (7.0711, -8.4289) -> (0, -1.3579)
  line L592 (0.5, 35.5) -> (20.5, 35.5)
  line L593 (20.5, 35.5) -> (20.5, 27.5)
  line L594 (20.5, 27.5) -> (0.5, 27.5)
  line L595 (0.5, 27.5) -> (0.5, 35.5)
  circle A9 centre (17.75, 31.5) radius 1.75
  circle A10 centre (12.9167, 31.5) radius 1.75
  circle A11 centre (8.0833, 31.5) radius 1.75
  circle A12 centre (3.25, 31.5) radius 1.75
  line L596 (-3.5, -36.5) -> (3.5, -36.5)
  line L597 (3.5, -36.5) -> (3.5, -31.5)
  line L598 (3.5, -31.5) -> (-3.5, -31.5)
  line L599 (-3.5, -31.5) -> (-3.5, -36.5)
  point P0 (0, 0)
  dimension "d10" = 2.44
  dimension "d11" = 2.44
  dimension "d12" = 2
  dimension "d13" = 12
  dimension "d14" = 0.64
  dimension "d15" = 0.64
  dimension "d18" = 2.54
  dimension "d21" = 2.54
  dimension "d26" = 12
  dimension "d33" = 2.54
  dimension "d36" = 2.54
  dimension "d41" = 12
  dimension "d46" = 10
  dimension "d47" = 135
  dimension "d48" = 21
  dimension "d49" = 20
  dimension "d50" = 8
  dimension "d51" = 8
  dimension "d52" = 1
  dimension "d53" = 3.5
  dimension "d54" = 2.75
  dimension "d57" = 4.8333
  dimension "d62" = 4
  dimension "d63" = 7
  dimension "d64" = 5
  constraints: 1192 end point, 10 parallel, 9 horizontal, 8 symmetric about line, 7 vertical, 5 perpendicular, 4 centre point, 3 point on line, 1 equal length, 1143 other
  measures "d10" distance of L6.end L5.end
  measures "d11" distance of L5.end L4.end
  measures "d12" distance between parallel lines of L2 L5
  measures "d13" distance from line of A2.centre L4
  measures "d14" distance of L12.end L11.end
  measures "d15" distance of L11.end L10.end
  measures "d18" distance of L4.start L14.start
  measures "d21" distance of L4.start L38.start
  measures "d26" distance of L30.start L128.start
  measures "d33" distance of L301.end L309.end
  measures "d36" distance of L301.end L333.end
  measures "d41" distance of L387.start L489.end
  measures "d46" distance of L587.start L587.end
  measures "d47" angle of L588 L587
  measures "d48" distance from line of L1 L587.start
  measures "d49" distance of L593.end L594.end
  measures "d50" distance of L592.end L593.end
  measures "d51" distance between parallel lines of L2 L593
  measures "d52" distance between parallel lines of L3 L592
  measures "d53" diameter of A9
  measures "d54" distance from line of L593 A9.centre
  measures "d57" distance of A9.centre A10.centre
  measures "d62" distance from line of L594 A9.centre
  measures "d63" distance of L598.end L597.end
  measures "d64" distance of L597.end L596.end
extrude "Extrusion2" add sketch "Sketch2" along normal blind 8.5 contours L13 L12 L11 L10 | L21 L20 L19 L18 | L29 L28 L27 L26 | L37 L36 L35 L34 | L45 L44 L43 L42 | L53 L52 L51 L50 | L61 L60 L59 L58 | L69 L68 L67 L66 | L77 L76 L75 L74 | L85 L84 L83 L82 | L93 L92 L91 L90 | L101 L100 L99 L98 | L111 L110 L109 L108 | L119 L118 L117 L116 | L127 L126 L125 L124 | L135 L134 L133 L132 | L143 L142 L141 L140 | L151 L150 L149 L148 | L159 L158 L157 L156 | L167 L166 L165 L164 | L175 L174 L173 L172 | L183 L182 L181 L180 | L191 L190 L189 L188 | L199 L198 L197 L196 | L209 L208 L207 L206 | L217 L216 L215 L214 | L225 L224 L223 L222 | L233 L232 L231 L230 | L241 L240 L239 L238 | L249 L248 L247 L246 | L257 L256 L255 L254 | L265 L264 L263 L262 | L273 L272 L271 L270 | L281 L280 L279 L278 | L289 L288 L287 L286 | L297 L296 L295 L294 | L303 L304 L305 L306 | L311 L312 L313 L314 | L319 L320 L321 L322 | L327 L328 L329 L330 | L335 L336 L337 L338 | L343 L344 L345 L346 | L351 L352 L353 L354 | L359 L360 L361 L362 | L367 L368 L369 L370 | L375 L376 L377 L378 | L383 L384 L385 L386 | L391 L392 L393 L394 | L399 L400 L401 L402 | L404 L405 L406 L410 | L412 L413 L414 L418 | L420 L421 L422 L426 | L428 L429 L430 L434 | L436 L437 L438 L442 | L444 L445 L446 L450 | L452 L453 L454 L458 | L460 L461 L462 L466 | L468 L469 L470 L474 | L476 L477 L478 L482 | L484 L485 L486 L490 | L495 L496 L497 L498 | L500 L501 L502 L506 | L508 L509 L510 L514 | L516 L517 L518 L522 | L524 L525 L526 L530 | L532 L533 L534 L538 | L540 L541 L542 L546 | L548 L549 L550 L554 | L556 L557 L558 L562 | L564 L565 L566 L570 | L572 L573 L574 L578 | L580 L581 L582 L586
extrude "Extrusion3" add sketch "Sketch2" along normal blind 2.5 contours L7 L6 L5 L4 | L17 L16 L15 L14 | L25 L24 L23 L22 | L33 L32 L31 L30 | L105 L104 L103 L102 | L114 L115 L113 L112 | L122 L123 L121 L120 | L130 L131 L129 L128 | L203 L202 L201 L200 | L212 L213 L211 L210 | L220 L221 L219 L218 | L228 L229 L227 L226 | L299 L300 L301 L302 | L307 L308 L309 L310 | L315 L316 L317 L318 | L323 L324 L325 L326 | L395 L396 L397 L398 | L403 L409 L407 L408 | L411 L417 L415 L416 | L419 L425 L423 L424 | L491 L492 L493 L494 | L499 L505 L503 L504 | L507 L513 L511 L512 | L515 L521 L519 L520
extrude "Extrusion4" add sketch "Sketch2" along normal blind 2.5 contours L41 L40 L39 L38 | L49 L48 L47 L46 | L57 L56 L55 L54 | L65 L64 L63 L62 | L138 L139 L137 L136 | L146 L147 L145 L144 | L154 L155 L153 L152 | L162 L163 L161 L160 | L236 L237 L235 L234 | L244 L245 L243 L242 | L252 L253 L251 L250 | L260 L261 L259 L258 | L331 L332 L333 L334 | L339 L340 L341 L342 | L347 L348 L349 L350 | L355 L356 L357 L358 | L427 L433 L431 L432 | L435 L441 L439 L440 | L443 L449 L447 L448 | L451 L457 L455 L456 | L523 L529 L527 L528 | L531 L537 L535 L536 | L539 L545 L543 L544 | L547 L553 L551 L552
extrude "Extrusion5" add sketch "Sketch2" along normal blind 2.5 contours L73 L72 L71 L70 | L81 L80 L79 L78 | L89 L88 L87 L86 | L97 L96 L95 L94 | L170 L171 L169 L168 | L178 L179 L177 L176 | L186 L187 L185 L184 | L194 L195 L193 L192 | L268 L269 L267 L266 | L276 L277 L275 L274 | L284 L285 L283 L282 | L292 L293 L291 L290 | L363 L364 L365 L366 | L371 L372 L373 L374 | L379 L380 L381 L382 | L387 L388 L389 L390 | L459 L465 L463 L464 | L467 L473 L471 L472 | L475 L481 L479 L480 | L483 L489 L487 L488 | L555 L561 L559 L560 | L563 L569 L567 L568 | L571 L577 L575 L576 | L579 L585 L583 L584
extrude "Extrusion6" add sketch "Sketch2" along normal blind 1.5 contours L587 L589 L591 L590
extrude "Extrusion7" add sketch "Sketch2" along normal blind 10 contours L592 L593 L594 L595 | A9 | A10 | A11 | A12
chamfer "Chamfer1" distance 1.5 distance2 5 1 edges at (10.5, 11, -35.5) measured on face at (7.1667, 11, -32.8333)
chamfer "Chamfer2" distance 1.5 distance2 8 1 edges at (10.5, 11, -27.5) measured on face at (7.1667, 11, -31.8333)
extrude "Extrusion8" add sketch "Sketch2" along normal blind 2 contours L599 L598 L597 L1
extrude "Extrusion9" cut sketch "Sketch2" along normal blind 19.25 contours A9 | A10 | A11 | A12
body "Solid1"
